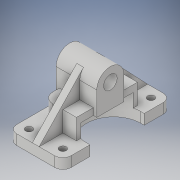
# Autodesk Inventor part: Part2019
Saved by Autodesk Inventor 2019 (Build 230136000, 136)
## iProperties
Created: 2026-04-19
Part Number: Part2019
Material: Generic
Document SubType Name: Modeling
Designer: 1
Density: 1 g/cm^3
Appearance: Default
Author: 1
Autodesk Inventor part; units mm, degrees
ref_plane "YZ Plane" through (0, 0, 0) normal (1, 0, 0) x (0, 1, 0)
ref_plane "XZ Plane" through (0, 0, 0) normal (0, 1, 0) x (-1, 0, 0)
ref_plane "XY Plane" through (0, 0, 0) normal (0, 0, 1) x (1, 0, 0)
sketch "Sketch4" plane through (0, 0, 0) normal (0, 1, 0) x (-1, 0, 0)
  line L0 (40, 80) -> (-40, 80)
  line L1 (-40, 80) -> (-40, -80)
  line L2 (-40, -80) -> (40, -80)
  line L3 (40, -80) -> (40, 80)
  line L4 (40, 80) -> (-40, -80) construction
  line L5 (-40, 80) -> (40, -80) construction
  point P0 (0, 0)
  dimension "d0" = 80
  dimension "d1" = 160
  constraints: 12 end point, 2 midpoint, 2 parallel, 1 horizontal, 1 perpendicular
  measures "d0" distance of L2.end L1.end
  measures "d1" distance of L1.end L0.end
extrude "Extrusion1" add sketch "Sketch4" along normal blind 15
sketch "Sketch5" plane through (0, 15, 0) normal (0, 1, 0) x (1, 0, 0)
  line L0 (-25, -45) -> (25, -45)
  line L1 (25, -45) -> (25, 45)
  line L2 (25, 45) -> (-25, 45)
  line L3 (-25, 45) -> (-25, -45)
  line L4 (-25, -45) -> (25, 45) construction
  line L5 (25, -45) -> (-25, 45) construction
  point P0 (0, 0)
  dimension "d4" = 50
  dimension "d5" = 90
  constraints: 12 end point, 2 midpoint, 2 parallel, 1 horizontal, 1 perpendicular
  measures "d4" distance of L2.end L1.end
  measures "d5" distance of L1.end L0.end
extrude "Extrusion2" add sketch "Sketch5" along normal blind 30
sketch "Sketch6" plane through (0, 15, 0) normal (0, 1, 0) x (1, 0, 0)
  point P0 (0, 0)
sketch "Sketch7" plane through (0, 0, 0) normal (1, 0, 0) x (0, 1, 0)
  line L0 (15, -80) -> (15, 80) projected
  line L1 (15, 0) -> (15, -20)
  line L2 (15, 0) -> (15, 20)
  line L3 (15, 20) -> (70, 20)
  line L4 (15, -20) -> (70, -20)
  arc A0 (70, -20) -> (70, 20) centre (70, 0) ccw
  point P0 (0, 0)
  dimension "d8" = 20
  dimension "d9" = 20
  dimension "d10" = 55
  dimension "d11" = 55
  constraints: 8 end point, 2 point on circle, 2 point on line, 1 centre point, 1 horizontal, 1 midpoint, 1 perpendicular
  measures "d8" distance of L1.start L1.end
  measures "d9" distance of L1.start L2.end
  measures "d10" distance of L2.end L3.end
  measures "d11" distance of L1.end L4.end
extrude "Extrusion3" add sketch "Sketch7" along normal blind 30 and the other way blind 30
sketch "Sketch8" plane through (0, 0, 0) normal (1, 0, 0) x (0, 1, 0)
  line L0 (15, 80) -> (83.7931, 14.4828)
  arc A0 (70, -20) -> (70, 20) centre (70, 0) ccw projected
  point P0 (0, 0)
  constraints: 2 end point, 1 point on circle, 1 tangent
extrude "Rib1" add sketch "Sketch8" along normal mid plane 10 rib yes fills toward (49.3621, 47.2052) open curves L0
mirror "Mirror1" about plane through (0, 0, 0) normal (0, 0, 1) of "Rib1"
sketch "Sketch9" plane through (0, 0, 0) normal (0, -1, 0) x (1, 0, 0)
  line L0 (40, 80) -> (40, -80) projected
  line L1 (40, 0) -> (40, -40)
  line L2 (40, 0) -> (40, 40)
  line L3 (40, 40) -> (35, 40)
  line L4 (40, -40) -> (35, -40)
  arc A0 (35, 40) -> (35, -40) centre (35, 0) ccw
  point P0 (0, 0)
  dimension "d22" = 40
  dimension "d23" = 40
  dimension "d24" = 5
  dimension "d25" = 5
  constraints: 8 end point, 2 point on circle, 2 point on line, 1 centre point, 1 horizontal, 1 midpoint, 1 perpendicular
  measures "d22" distance of L1.start L1.end
  measures "d23" distance of L1.start L2.end
  measures "d24" distance of L2.end L3.end
  measures "d25" distance of L1.end L4.end
extrude "Extrusion4" cut sketch "Sketch9" against normal blind 35
sketch "Sketch10" plane through (30, 0, 0) normal (1, 0, 0) x (0, 0, -1)
  arc A0 (20, 70) -> (-20, 70) centre (0, 70) ccw projected
  circle A1 centre (0, 70) radius 10
  point P0 (0, 0)
  dimension "d28" = 20
  constraints: 1 centre point, 1 coincident
  measures "d28" diameter of A1
extrude "Extrusion5" cut sketch "Sketch10" against normal blind 60
fillet "Fillet1" radius 12 4 edges at (40, 7.5, -80) (40, 7.5, 80) (-40, 7.5, 80) (-40, 7.5, -80)
fillet "Fillet2" radius 15 2 edges at (-25, 30, 45) (-25, 30, -45)
sketch "Sketch12" plane through (0, 15, 0) normal (0, 1, 0) x (1, 0, 0)
  arc A0 (-40, -68) -> (-28, -80) centre (-28, -68) ccw projected
  line L0 (-40, 68) -> (-40, -68) projected
  circle A1 centre (-25, -65) radius 5
  point P0 (0, 0)
  dimension "d41" = 10
  constraints: 1 centre point
  measures "d41" diameter of A1
extrude "Extrusion7" cut sketch "Sketch12" against normal blind 15
mirror "Mirror4" about plane through (0, 0, 0) normal (0, 0, 1) of "Extrusion7"
mirror "Mirror5" about plane through (0, 0, 0) normal (1, 0, 0) of "Extrusion7", "Mirror4"
body "Solid1"
